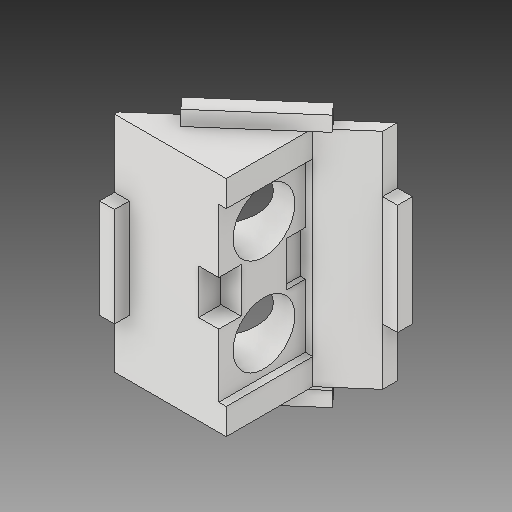
# Autodesk Inventor part: Sensor
Saved by Autodesk Inventor 2019 (Build 230136000, 136)
## iProperties
Created: 2020-12-06
Part Number: Sensor
Material: Пластик АБС
Document SubType Name: Modeling
Designer: Professional
Density: 1.06 g/cm^3
Appearance: Гладкий — белый
Author: Professional
Autodesk Inventor part; units mm, degrees
ref_plane "YZ Plane" through (0, 0, 0) normal (1, 0, 0) x (0, 1, 0)
ref_plane "XZ Plane" through (0, 0, 0) normal (0, 1, 0) x (-1, 0, 0)
ref_plane "XY Plane" through (0, 0, 0) normal (0, 0, 1) x (1, 0, 0)
sketch "Эскиз1" plane through (0, 0, 0) normal (0, 1, 0) x (-1, 0, 0)
  line L0 (0, -4) -> (0, 0)
  line L1 (40, 31) -> (10, 31)
  line L2 (40, 31) -> (0, -4)
  line L3 (10, 31) -> (10, 8.75)
  line L4 (10, 8.75) -> (0, 0)
  dimension "d2" = 35
  dimension "d3" = 40
  dimension "d4" = 30
  dimension "d5" = 4
  dimension "d6" = 22.25
  constraints: 10 end point, 2 vertical, 1 horizontal, 1 parallel
  measures "d2" vertical distance of L1.start L0.start
  measures "d3" horizontal distance of L1.start L0.end
  measures "d4" distance of L1.start L1.end
  measures "d5" distance of L0.start L0.end
  measures "d6" distance of L1.end L3.end
extrude "Выдавливание1" add sketch "Эскиз1" along normal blind 60
sketch "Эскиз2" plane through (-10, 0, 31) normal (1, 0, 0) x (0, 0, -1)
  line L0 (0, 0) -> (0, 60) projected
  line L1 (22.25, 0) -> (22.25, 60) projected
  line L2 (0, 53) -> (22.25, 53)
  line L3 (22.25, 53) -> (22.25, 7)
  line L4 (22.25, 7) -> (0, 7)
  line L5 (0, 7) -> (0, 53)
  point P0 (31, 0)
  point P1 (0, 30)
  dimension "d9" = 46
  constraints: 8 end point, 2 midpoint, 2 parallel, 2 point on line, 1 horizontal, 1 perpendicular
  measures "d9" distance between parallel lines of L4 L2
extrude "Выдавливание2" cut sketch "Эскиз2" against normal blind 2
sketch "Эскиз3" plane through (-12, 0, 31) normal (1, 0, 0) x (0, 0, -1)
  circle A0 centre (11.125, 43) radius 8.3
  circle A1 centre (11.125, 17) radius 8.3
  line L0 (11.125, 17) -> (11.125, 43) construction
  line L1 (0, 7) -> (0, 53) projected
  line L2 (0, 53) -> (22.25, 53) projected
  point P0 (31, 0)
  point P1 (11.125, 30)
  point P2 (0, 30)
  point P3 (11.125, 53)
  dimension "d12" = 16.6
  dimension "d13" = 26
  constraints: 3 midpoint, 2 centre point, 2 end point, 1 equal radius, 1 horizontal alignment, 1 vertical, 1 vertical alignment
  measures "d12" diameter of A0
  measures "d13" distance of L0.start L0.end
extrude "Выдавливание3" cut sketch "Эскиз3" against normal through all
sketch "Эскиз4" plane through (-12, 0, 31) normal (1, 0, 0) x (0, 0, -1)
  line L0 (22.25, 53) -> (22.25, 7) projected
  line L1 (17.25, 36) -> (22.25, 36)
  line L2 (22.25, 36) -> (22.25, 24)
  line L3 (22.25, 24) -> (17.25, 24)
  line L4 (17.25, 24) -> (17.25, 36)
  line L5 (0, 36) -> (5, 36)
  line L6 (5, 36) -> (5, 24)
  line L7 (5, 24) -> (0, 24)
  line L8 (0, 24) -> (0, 36)
  line L9 (0, 7) -> (0, 53) projected
  point P0 (31, 0)
  point P1 (0, 30)
  dimension "d16" = 5
  dimension "d17" = 12
  constraints: 16 end point, 4 parallel, 4 point on line, 2 horizontal, 2 midpoint, 2 perpendicular, 1 collinear
  measures "d16" distance between parallel lines of L0 L4
  measures "d17" distance between parallel lines of L1 L3
extrude "Выдавливание4" cut sketch "Эскиз4" against normal blind 1.4
sketch "Эскиз5" plane through (0, 0, 0) normal (1, 0, 0) x (0, 0, -1)
  line L0 (4, 0) -> (4, 60) projected
  line L1 (0, 44.8) -> (4, 44.8)
  line L2 (4, 44.8) -> (4, 15.2)
  line L3 (4, 15.2) -> (0, 15.2)
  line L4 (0, 15.2) -> (0, 44.8)
  line L5 (0, 0) -> (0, 60) projected
  point P0 (4, 30)
  dimension "d20" = 29.6
  constraints: 8 end point, 2 midpoint, 2 parallel, 2 point on line, 1 horizontal, 1 perpendicular
  measures "d20" distance between parallel lines of L1 L3
extrude "Выдавливание5" add sketch "Эскиз5" along normal blind 4
sketch "Эскиз6" plane through (-40, 0, 31) normal (0, 0, 1) x (1, 0, 0)
  line L0 (0, 0) -> (0, 60) projected
  line L1 (0, 15.2) -> (4, 15.2)
  line L2 (4, 15.2) -> (4, 41.8)
  line L3 (4, 41.8) -> (0, 41.8)
  line L4 (0, 41.8) -> (0, 15.2)
  point P0 (40, 0)
  point P1 (0, 30)
  dimension "d23" = 4
  dimension "d24" = 26.6
  dimension "d37" = 14.8
  constraints: 8 end point, 2 parallel, 1 horizontal, 1 midpoint, 1 perpendicular, 1 point on line
  measures "d23" distance between parallel lines of L0 L2
  measures "d24" distance between parallel lines of L1 L3
  measures "d37" distance from line of L1 point (0, 30)
extrude "Выдавливание6" add sketch "Эскиз6" along normal blind 5
sketch "Эскиз7" plane through (0, 0, 0) normal (0, -1, 0) x (1, 0, 0)
  line L0 (-9.1664, 4.0206) -> (-6.5324, 7.0309)
  line L1 (-10, 8.75) -> (0, 0) projected
  line L2 (0, -4) -> (-40, 31) projected
  line L3 (-9.1664, 4.0206) -> (-30.8406, 22.9855)
  line L4 (-17.8, 11.575) -> (-36.7714, 28.175) projected
  line L5 (-30.8406, 22.9855) -> (-28.2066, 25.9958)
  line L6 (-28.2066, 25.9958) -> (-6.5324, 7.0309)
  dimension "d28" = 4
  dimension "d29" = 28.8
  dimension "d30" = 12.18
  constraints: 9 end point, 2 perpendicular, 2 point on line, 1 parallel
  measures "d28" distance between parallel lines of L2 L6
  measures "d29" distance between parallel lines of L5 L0
  measures "d30" distance from line of L2.start L0
extrude "Выдавливание7" add sketch "Эскиз7" along normal blind 4
sketch "Эскиз8" plane through (0, 60, 0) normal (0, 1, 0) x (1, 0, 0)
  line L0 (-9.1664, -4.0206) -> (-6.5324, -7.0309) projected
  line L1 (-6.5324, -7.0309) -> (-28.2066, -25.9958) projected
  line L2 (-28.2066, -25.9958) -> (-30.8406, -22.9855) projected
  line L3 (-30.8406, -22.9855) -> (-9.1664, -4.0206) projected
  point P0 (0, 0)
extrude "Выдавливание8" add sketch "Эскиз8" along normal blind 4
sketch "Эскиз9" plane through (-40, 0, 31) normal (0, 0, 1) x (1, 0, 0)
  line L0 (0, 41.8) -> (4, 41.8) projected
  line L1 (4, 41.8) -> (4, 15.2) projected
  line L2 (4, 15.2) -> (0, 15.2) projected
  line L3 (0, 0) -> (0, 15.2) projected
  line L4 (0, 0) -> (30, 0) projected
  line L5 (30, 0) -> (30, 7) projected
  line L6 (30, 7) -> (28, 7) projected
  line L7 (28, 7) -> (28, 24) projected
  line L8 (28, 24) -> (26.6, 24) projected
  line L9 (26.6, 24) -> (26.6, 36) projected
  line L10 (26.6, 36) -> (28, 36) projected
  line L11 (28, 36) -> (28, 53) projected
  line L12 (28, 53) -> (30, 53) projected
  line L13 (30, 53) -> (30, 60) projected
  line L14 (0, 60) -> (30, 60) projected
  line L15 (0, 41.8) -> (0, 60) projected
  point P0 (40, 0)
extrude "Выдавливание9" add sketch "Эскиз9" along normal blind 1
sketch "Эскиз10" plane through (-13.4, 0, 31) normal (1, 0, 0) x (0, 0, -1)
  line L0 (5, 24) -> (-1, 24) projected
  line L1 (5, 36) -> (5, 24) projected
  line L2 (-1, 36) -> (5, 36) projected
  line L3 (-1, 24) -> (-1, 36) projected
  point P0 (31, 0)
extrude "Выдавливание10" cut sketch "Эскиз10" against normal blind 4
